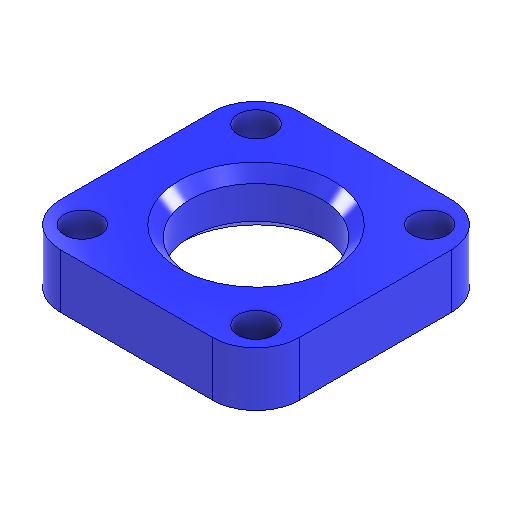
# Autodesk Inventor part: Chumacera
Saved by Autodesk Inventor 2025.3 (Build 293356000, 356)
## iProperties
Created: 2025-10-28
Part Number: Chumacera
Material: ABS Plastic
Document SubType Name: Modeling
Designer: Gabriel Bojaca
Density: 1.06 g/cm^3
Appearance: Blue - Wall Paint - Glossy
Author: Gabriel Bojaca
Autodesk Inventor part; units mm, degrees
ref_plane "YZ Plane" through (0, 0, 0) normal (1, 0, 0) x (0, 1, 0)
ref_plane "XZ Plane" through (0, 0, 0) normal (0, 1, 0) x (-1, 0, 0)
ref_plane "XY Plane" through (0, 0, 0) normal (0, 0, 1) x (1, 0, 0)
sketch "Sketch1" plane through (0, 0, 0) normal (0, 1, 0) x (-1, 0, 0)
  line L0 (-8, -8) -> (8, -8) construction
  line L1 (8, -8) -> (8, 8) construction
  line L2 (8, 8) -> (-8, 8) construction
  line L3 (-8, 8) -> (-8, -8) construction
  line L4 (-8, -8) -> (8, 8) construction
  line L5 (8, -8) -> (-8, 8) construction
  circle A0 centre (-8, 8) radius 1.65
  line L6 (0, 0) -> (0, 2.722) construction
  line L7 (0, 2.722) -> (0, 0) construction
  line L8 (-3.7265, 0) -> (0, 0) construction
  circle A1 centre (8, 8) radius 1.65
  line L9 (8, -8) -> (-8, -8) construction
  circle A2 centre (-8, -8) radius 1.65
  circle A3 centre (8, -8) radius 1.65
  line L10 (-11, -11) -> (11, -11)
  line L11 (11, -11) -> (11, 11)
  line L12 (11, 11) -> (-11, 11)
  line L13 (-11, 11) -> (-11, -11)
  line L14 (-11, -11) -> (11, 11) construction
  line L15 (11, -11) -> (-11, 11) construction
  circle A4 centre (0, 0) radius 6.05
  dimension "d0" = 16
  dimension "d1" = 16
  dimension "d2" = 3.3
  dimension "d3" = 22
  dimension "d4" = 22
  dimension "d5" = 12.1
  constraints: 32 end point, 5 centre point, 5 equal length, 4 midpoint, 3 coincident, 3 perpendicular, 3 symmetric about line, 2 horizontal, 1 vertical, 3 other
  measures "d0" distance of L2.end L1.end
  measures "d1" distance of L1.end L0.end
  measures "d2" diameter of A0
  measures "d3" distance of L12.end L11.end
  measures "d4" distance of L11.end L10.end
  measures "d5" diameter of A4
extrude "Extrusion1" add sketch "Sketch1" along normal blind 5
fillet "Fillet1" radius 4 4 edges at (-11, 2.5, -11) (-11, 2.5, 11) (11, 2.5, 11) (11, 2.5, -11)
chamfer "Chamfer1" distance 1 angle 45 2 edges at (6.05, 5, 0) (6.05, 0, 0)
body "Solid1"
